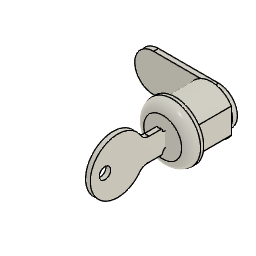
Key Assy v21 (Autodesk Fusion 360 archive; units mm, degrees)
design "Defender Security 5/16 in key Cabinet and Drawer Lock"
Autodesk Fusion 360 part; units mm, degrees
sketch "Sketch1" plane through (0, 0, 0) normal (0, 1, 0) x (1, 0, 0) in component "Shaft"
  circle A0 centre (0, 0) radius 11.43
  dimension "d1" = 22.86
  constraint coincident A0.centre origin
  measures "d1" diameter of A0
extrude "Extrude1" add sketch "Sketch1" against normal blind 5.08 makes body 1 in component "Shaft"
fillet "Fillet1" radius 3.81 1 edges at (-10.6565, -5.08, -4.1333) on bodies 1 in component "Shaft"
sketch "Sketch2" plane through (0, 0, 0) normal (0, 1, 0) x (-1, 0, 0) in component "Shaft"
  circle A0 centre (0, 0) radius 11.43
  circle A1 centre (0, 0) radius 9.525
  line L0 (8.0645, -16.137) -> (-8.0645, -16.137)
  line L1 (-8.0645, -16.137) -> (-8.0645, 16.137)
  line L2 (-8.0645, 16.137) -> (8.0645, 16.137)
  line L3 (8.0645, 16.137) -> (8.0645, -16.137)
  line L4 (8.0645, -16.137) -> (-8.0645, 16.137) construction
  line L5 (-8.0645, -16.137) -> (8.0645, 16.137) construction
  dimension "d6" = 19.05
  dimension "d7" = 16.129
  constraint coincident A0.centre A1.centre
  constraint horizontal L0
  constraint perpendicular L0 L1
  constraint parallel L0 L2
  constraint parallel L1 L3
  constraint coincident L4 A0.centre
  constraint coincident L5 A0.centre
  measures "d6" diameter of A1
  measures "d7" distance of L1.end L2.end
extrude "Extrude2" add sketch "Sketch2" along normal blind 14.478 contours A1 L1 L3 bodies 1 in component "Shaft"
copy_body "CutPasteBodies1" bodies 1 removing the originals makes body 2 in component "Shaft"
sketch "Sketch1 (2)" plane through (0, 14.478, 0) normal (0, 1, 0) x (-1, 0, 0) in component "Arm"
  arc A0 (-8.0645, -5.0685) -> (8.0645, -5.0685) centre (0, 0) ccw
  line L0 (8.0645, -5.0685) -> (8.0645, 5.0685)
  arc A1 (8.0645, 5.0685) -> (-8.0645, 5.0685) centre (0, 0) ccw
  line L1 (-8.0645, 5.0685) -> (-8.0645, -5.0685)
  line L2 (0, 7.5565) -> (24.1935, 7.5565)
  line L3 (0, -7.5565) -> (24.1935, -7.5565)
  arc A2 (24.1935, -7.5565) -> (24.1935, 7.5565) centre (24.1935, 0) ccw
  arc A3 (0, 7.5565) -> (0, -7.5565) centre (0, 0) ccw
  line L4 (4.3815, 4.3815) -> (-4.3815, 4.3815)
  line L5 (-4.3815, 4.3815) -> (-4.3815, -4.3815)
  line L6 (-4.3815, -4.3815) -> (4.3815, -4.3815)
  line L7 (4.3815, -4.3815) -> (4.3815, 4.3815)
  line L8 (4.3815, 4.3815) -> (-4.3815, -4.3815) construction
  line L9 (-4.3815, 4.3815) -> (4.3815, -4.3815) construction
  dimension "d11" = 15.113
  dimension "d12" = 31.75
  dimension "d13" = 8.763
  constraint coincident A0.centre A1.centre
  constraint equal A2 A3
  constraint tangent L2 A2
  constraint horizontal L2
  constraint tangent L3 A2
  constraint parallel L2 L3
  constraint horizontal L4
  constraint perpendicular L4 L5
  constraint parallel L4 L6
  constraint parallel L5 L7
  constraint coincident L8 A0.centre
  constraint coincident L9 A0.centre
  constraint equal L6 L7
  measures "d11" diameter of A2
  measures "d13" distance of L5.end L6.end
extrude "Extrude1'" add sketch "Sketch1 (2)" along normal blind 1.9812 separate body contours A0 L0 A1 L2 L3 A3 | A0 L0 A1 L2 L3 A2 makes body 3 in component "Arm"
sketch "Sketch2 (2)" plane through (0, 0, 0) normal (1, 0, 0) x (0, 1, 0) in component "Key"
  arc A0 (12.9212, 3.491) -> (12.4132, 3.999) centre (12.4132, 3.491) ccw
  arc A1 (12.9212, 3.1831) -> (13.4292, 2.6751) centre (13.4292, 3.1831) ccw
  arc A2 (27.7358, -2.8772) -> (28.1431, -2.6728) centre (27.7358, -2.3692) ccw
  line L0 (27.7358, -2.8772) -> (15.2072, -2.8772)
  line L1 (13.4292, 2.6751) -> (28.2966, 2.6751)
  line L2 (12.9212, 3.1831) -> (12.9212, 3.491)
  arc A3 (12.479, -5.0685) -> (12.975, -4.6701) centre (12.479, -4.5605) ccw
  line L3 (30.1607, 0.0345) -> (28.1431, -2.6728)
  arc A4 (4.3127, 5.8054) -> (3.7719, -6.6005) centre (-5.077, 0) ccw
  line L4 (28.6939, 2.4836) -> (30.1508, 0.6545)
  line L5 (6.8259, -5.0685) -> (12.479, -5.0685)
  arc A5 (15.2072, -2.8772) -> (12.975, -4.6701) centre (15.2072, -5.1632) ccw
  arc A6 (28.6939, 2.4836) -> (28.2966, 2.6751) centre (28.2966, 2.1671) ccw
  line L6 (12.9212, -5.0685) -> (12.9212, -5.1632)
  line L7 (12.4132, 3.999) -> (7.5533, 3.999)
  arc A7 (30.1607, 0.0345) -> (30.1508, 0.6545) centre (29.7534, 0.338) ccw
  circle A8 centre (-10.2031, 0) radius 2.286
  arc A9 (4.3127, 5.8054) -> (7.5533, 3.999) centre (7.5533, 7.809) ccw
  arc A10 (6.8259, -5.0685) -> (3.7719, -6.6005) centre (6.8259, -8.8785) ccw
  dimension "d24" = 2.286
  dimension "d25" = 0.508
  dimension "d26" = 4.572
  dimension "d29" = 3.81
  constraint horizontal L7
  constraint horizontal L5
  constraint vertical L6
  constraint horizontal L1
  constraint horizontal L0
  constraint tangent A5 L6
  constraint tangent L0 A5
  constraint perpendicular L2 L7
  constraint tangent A1 L2
  constraint tangent A1 L1
  constraint tangent A0 L7
  constraint tangent A0 L2
  constraint equal A0 A1
  constraint tangent A3 L5
  constraint tangent A3 A5
  constraint equal A1 A3
  constraint tangent L1 A6
  constraint tangent L4 A6
  constraint equal A1 A6
  constraint tangent A2 L3
  constraint tangent A2 L0
  constraint equal A1 A2
  constraint tangent L4 A7
  constraint tangent L3 A7
  constraint equal A1 A7
  constraint tangent A4 A9
  constraint tangent L7 A9
  constraint tangent A4 A10
  constraint tangent L5 A10
  constraint equal A9 A10
  measures "d24" radius of A5
  measures "d25" radius of A1
  measures "d26" diameter of A8
  measures "d29" radius of A9
extrude "Extrude2'" add sketch "Sketch2 (2)" along normal mid plane 1.8796 separate body makes body 4 in component "Key"
move_body "Move1" bodies 4 to x (1, 0, 0) y (0, 1, 0) z (0, 0, 1) at (0, -19.05, 0) in component "Key"
component "Shaft" placed x (1, 0, 0) y (0, 1, 0) z (0, 0, 1) at (0, 0, 0)
component "Arm" placed x (1, 0, 0) y (0, -1, 0) z (0, 0, -1) at (0, 31.877, 0)
component "Key" placed x (1, 0, 0) y (0, 1, 0) z (0, 0, 1) at (0, 0, 0)
equation "d8 = LockLength"
equation "LockLength = ( 0.57 ) * 1 in" comment "This is the distance measured by caliper from the lip of the key to the end of the key. This is also the \"advertised\" key length-.04 in."
